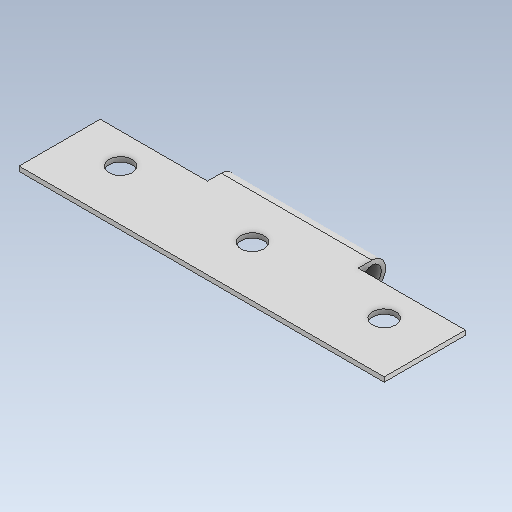
# Autodesk Inventor part: Ala 2 Bisagra tipo Libro Chica
Saved by Autodesk Inventor 2020 (Build 240168000, 168)
## iProperties
Created: 2020-06-20
Part Number: Ala 2 Bisagra tipo Libro Chica
Material: Genérico
Document SubType Name: Modeling
Designer: Pipi
Density: 1 g/cm^3
Appearance: Valor por defecto
Author: Pipi
Autodesk Inventor part; units mm, degrees
ref_plane "YZ Plane" through (0, 0, 0) normal (1, 0, 0) x (0, 1, 0)
ref_plane "XZ Plane" through (0, 0, 0) normal (0, 1, 0) x (-1, 0, 0)
ref_plane "XY Plane" through (0, 0, 0) normal (0, 0, 1) x (1, 0, 0)
sketch "Boceto1" plane through (0, 0, 0) normal (0, 1, 0) x (-1, 0, 0)
  line L0 (6.207, 40.007) -> (6.207, 26.007)
  line L1 (6.207, 26.007) -> (-56.793, 26.007)
  line L2 (-56.793, 26.007) -> (-56.793, 40.007)
  line L3 (-56.793, 40.007) -> (6.207, 40.007)
  circle A0 centre (-25.293, 31.257) radius 2
  circle A1 centre (-2.543, 31.257) radius 2
  circle A2 centre (-48.043, 31.257) radius 2
  point P0 (0, 0)
  point P1 (0, 0)
  dimension "d0" = 14
  dimension "d1" = 63
  dimension "d24" = 4
  dimension "d25" = 4
  dimension "d26" = 4
  dimension "d27" = 8.75
  dimension "d28" = 8.75
  dimension "d29" = 8.75
  dimension "d30" = 31.5
  dimension "d31" = 8.75
  dimension "d32" = 8.75
  constraints: 8 end point, 3 centre point, 3 perpendicular, 1 vertical
  measures "d0" distance of L0.start L0.end
  measures "d1" distance of L0.end L1.end
  measures "d24" diameter of A0
  measures "d25" diameter of A1
  measures "d26" diameter of A2
  measures "d27" distance from line of L0 A1.centre
  measures "d28" distance from line of L3 A1.centre
  measures "d29" distance from line of L3 A0.centre
  measures "d30" distance from line of L0 A0.centre
  measures "d31" distance from line of L2 A2.centre
  measures "d32" distance from line of L3 A2.centre
extrude "Extrusión1" add sketch "Boceto1" along normal blind 0.8
sketch "Boceto7" plane through (56.793, 0, 40.007) normal (1, 0, 0) x (0, 0, -1)
  circle A0 centre (16.375, -1.575) radius 2.375
  circle A1 centre (16.375, -1.575) radius 1.625
  line L0 (0, 0.8) -> (14, 0.8) projected
  line L1 (14, 0) -> (14, 0.8) projected
  line L2 (14, 0) -> (14, -1.575)
  line L3 (16.375, 0.8) -> (14, 0.8)
  line L4 (14, 0) -> (0, 0) projected
  line L5 (14, 0.8) -> (14, 0)
  point P0 (40.007, 0)
  dimension "d33" = 4.75
  dimension "d34" = 3.25
  constraints: 6 end point, 3 tangent, 2 centre point, 2 point on circle, 1 coincident, 1 horizontal, 1 perpendicular
  measures "d33" diameter of A0
  measures "d34" diameter of A1
extrude "Extrusión6" add sketch "Boceto7" against normal blind 44.5
sketch "Boceto9" plane through (56.793, 0, 40.007) normal (1, 0, 0) x (0, 0, -1)
  circle A0 centre (16.375, -1.575) radius 1.625 projected
  circle A1 centre (16.375, -1.575) radius 2.375
  line L0 (14, 0.8) -> (16.375, 0.8) projected
  line L1 (16.375, 0.8) -> (14, 0.8)
  line L2 (14, -1.575) -> (14, 0) projected
  line L3 (14, 0.8) -> (14, -1.575)
  point P0 (40.007, 0)
  constraints: 4 end point, 2 collinear, 2 tangent, 1 centre point, 1 coincident
extrude "Extrusión8" cut sketch "Boceto9" against normal blind 18.5 contours A0 | A1 | A1 L2 L3 L0
